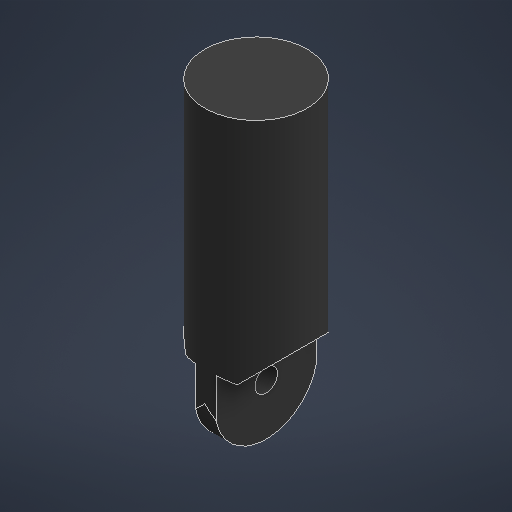
# Autodesk Inventor part: Camera encase
Saved by Autodesk Inventor 2026.2 (Build 302298010, 298A)
## iProperties
Created: 2026-04-02
Part Number: Camera encase
Material: Rubber
Document SubType Name: Modeling
Designer: piete
Density: 0.93 g/cm^3
Appearance: Rubber - Black
Author: piete
Autodesk Inventor part; units mm, degrees
ref_plane "YZ Plane" through (0, 0, 0) normal (1, 0, 0) x (0, 1, 0)
ref_plane "XZ Plane" through (0, 0, 0) normal (0, 1, 0) x (-1, 0, 0)
ref_plane "XY Plane" through (0, 0, 0) normal (0, 0, 1) x (1, 0, 0)
sketch "Sketch1" plane through (0, 0, 0) normal (0, 1, 0) x (-1, 0, 0)
  circle A0 centre (0, 0) radius 5
  dimension "d0" = 10
  constraints: 1 centre point, 1 coincident
  measures "d0" diameter of A0
extrude "Extrusion1" add sketch "Sketch1" along normal blind 20
sketch "Sketch2" plane through (0, 0, 0) normal (1, 0, 0) x (0, 1, 0)
  circle A0 centre (-5, 0) radius 1.1
  line L0 (0, -5) -> (0, 5) projected
  circle A1 centre (-5, 0) radius 5
  line L1 (0, 5) -> (-5, 5)
  line L2 (-5, -5) -> (0, -5)
  line L3 (0, -5) -> (0, 5)
  point P0 (0, 0)
  dimension "d3" = 2.2
  dimension "d4" = 5
  dimension "d5" = 5
  dimension "d6" = 10
  constraints: 6 end point, 2 centre point, 2 point on circle, 2 tangent, 1 coincident, 1 collinear
  measures "d3" diameter of A0
  measures "d4" distance from line of A0.centre L0
  measures "d5" horizontal distance of A0.centre L0.start
  measures "d6" diameter of A1
extrude "Extrusion2" add sketch "Sketch2" along normal mid plane 2
sketch "Sketch3" plane through (1, 0, 0) normal (1, 0, 0) x (0, 0, -1)
  circle A0 centre (0, -5) radius 1.1 projected
  line L0 (0, -5) -> (4.3301, -2.5)
  line L1 (0, -5) -> (5, -5) construction
  line L2 (0, -5) -> (-4.3301, -2.5)
  line L3 (0, -5) -> (5, -5) construction
  circle A1 centre (0, -5) radius 1.1
  circle A2 centre (0, -5) radius 5
  line L4 (0, -5) -> (5, -2.1132)
  line L5 (0, -5) -> (-5, -2.1132)
  line L6 (-5, 0) -> (-5, -5) projected
  line L7 (-5, 0) -> (-5, -2.1132)
  line L8 (5, -2.1132) -> (5, 0)
  line L9 (5, 0) -> (-5, 0)
  line L10 (4.899, 0) -> (-4.899, 0) projected
  point P0 (0, 0)
  point P1 (0, 0)
  dimension "d9" = 5
  dimension "d10" = 30
  dimension "d11" = 5
  dimension "d12" = 150
  dimension "d13" = 2.1132
  constraints: 18 end point, 2 centre point, 2 coincident, 2 collinear, 2 equal length, 2 horizontal, 2 point on line, 1 point on circle, 1 vertical
  measures "d9" distance of L0.start L0.end
  measures "d10" angle of L1 L0
  measures "d11" distance of L0.start L2.end
  measures "d12" angle of L3 L2
  measures "d13" distance of L4.end L8.end
extrude "Extrusion3" add sketch "Sketch3" along normal blind 5 contours A2 L9 L8 L4 | L5 L6 L9 A2
mirror "Mirror1" about plane through (0, 0, 0) normal (1, 0, 0) of "Extrusion3"
sketch "Sketch4" plane through (0, 20, 0) normal (0, 1, 0) x (1, 0, 0)
  circle A0 centre (0, 0) radius 5
  circle A1 centre (0, 0) radius 10
  dimension "d16" = 10
  dimension "d17" = 20
  constraints: 2 centre point, 2 coincident
  measures "d16" diameter of A0
  measures "d17" diameter of A1
extrude "Extrusion4" cut sketch "Sketch4" against normal through all
body "Solid1"
